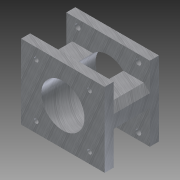
# Autodesk Inventor part: motor bracket GL-15N
Saved by Autodesk Inventor 2011 (Build 150239000, 239)
## iProperties
Created: 2014-01-21
Part Number: motor bracket GL-15N
Document SubType Name: Modeling
Designer: Devon
Density: 1 g/cm^3
Author: Devon
Autodesk Inventor part; units mm, degrees
ref_plane "YZ Plane" through (0, 0, 0) normal (1, 0, 0) x (0, 1, 0)
ref_plane "XZ Plane" through (0, 0, 0) normal (0, 1, 0) x (-1, 0, 0)
ref_plane "XY Plane" through (0, 0, 0) normal (0, 0, 1) x (1, 0, 0)
sketch "Sketch1" plane through (0, 0, 0) normal (0, 0, 1) x (1, 0, 0)
  line L0 (0, 0) -> (74, 0)
  line L1 (74, 0) -> (74, 66)
  line L2 (74, 66) -> (0, 66)
  line L3 (0, 66) -> (0, 0)
  line L4 (0, 0) -> (0, 9.43)
  line L5 (74, 0) -> (64.57, 0)
  line L6 (0, 66) -> (9.43, 66)
  line L7 (74, 66) -> (64.57, 66)
  line L8 (37, 33) -> (75, 33) construction
  line L9 (37, 33) -> (75, 33) construction
  circle A0 centre (10.1299, 59.8701) radius 2.5
  circle A1 centre (63.8701, 59.8701) radius 2.5
  circle A2 centre (63.8701, 6.1299) radius 2.5
  circle A3 centre (10.1299, 6.1299) radius 2.5
  dimension "d0" = 74
  dimension "d1" = 66
  dimension "d2" = 9.43
  dimension "d4" = 9.43
  dimension "d6" = 9.43
  dimension "d8" = 9.43
  dimension "d14" = 5
  dimension "d15" = 5
  dimension "d16" = 5
  dimension "d17" = 5
  constraints: 20 end point, 4 centre point, 4 point on line, 3 horizontal, 2 parallel, 1 perpendicular
  measures "d0" distance of L2.end L1.end
  measures "d1" distance of L1.end L0.end
  measures "d2" distance of L0.start L4.end
  measures "d4" distance of L0.end L5.end
  measures "d6" distance of L2.end L6.end
  measures "d8" distance of L1.end L7.end
  measures "d14" diameter of A0
  measures "d15" diameter of A1
  measures "d16" diameter of A2
  measures "d17" diameter of A3
extrude "Extrusion1" add sketch "Sketch1" along normal blind 8
sketch "Sketch2" plane through (0, 0, 8) normal (0, 0, 1) x (1, 0, 0)
  line L0 (0, 0) -> (0, 66) projected
  line L1 (74, 0) -> (0, 0) projected
  line L2 (74, 66) -> (74, 0) projected
  line L3 (5.4025, 46.4704) -> (0, 41.0679)
  line L4 (14.4661, 10.4661) -> (24.9321, 0)
  line L5 (68.5975, 46.4704) -> (74, 41.0679)
  line L6 (14.4661, 10.4661) -> (0, 24.9321)
  arc A0 (23.5296, 46.4704) -> (50.4704, 46.4704) centre (37, 33) ccw
  line L7 (50.4704, 46.4704) -> (68.5975, 46.4704)
  line L8 (23.5296, 46.4704) -> (5.4025, 46.4704)
  circle A1 centre (63.8701, 6.1299) radius 2.5 projected
  circle A2 centre (10.1299, 6.1299) radius 2.5 projected
  line L9 (57.1349, 12.8651) -> (74, 29.7303)
  line L10 (57.1349, 12.8651) -> (44.2697, 0)
  line L11 (10.1299, 6.1299) -> (16.8651, 12.8651)
  line L12 (16.8651, 12.8651) -> (0, 29.7303)
  line L13 (16.8651, 12.8651) -> (29.7303, 0)
  point P0 (49.0679, 0)
  point P1 (74, 24.9321)
  dimension "d23" = 38.1
  dimension "d26" = 9.525
  dimension "d27" = 9.525
  constraints: 22 end point, 10 point on line, 3 collinear, 2 perpendicular, 2 point on circle, 1 centre point
  measures "d23" diameter of A0
  measures "d26" distance of A1.centre L9.start
  measures "d27" distance of L11.start L11.end
extrude "Extrusion2" add sketch "Sketch2" along normal blind 32 contours L0 L3 L8 A0 L7 L5 L2 L9 L10 L1 L13 L12
sketch "Sketch4" plane through (0, 0, 40) normal (0, 0, 1) x (1, 0, 0)
  line L0 (0, 0) -> (74, 0)
  line L1 (74, 0) -> (74, 65.908)
  line L2 (74, 65.908) -> (0, 65.908)
  line L3 (0, 65.908) -> (0, 0)
  line L4 (4, 65.908) -> (70, 65.908)
  line L5 (70, 0) -> (4, 0)
  line L6 (4, 65.908) -> (13.43, 65.908)
  line L7 (13.43, 65.908) -> (13.43, 56.478)
  line L8 (4, 9.43) -> (13.43, 9.43)
  line L9 (70, 0) -> (60.57, 0)
  line L10 (60.57, 0) -> (60.57, 9.43)
  line L11 (70, 65.908) -> (60.57, 65.908)
  line L12 (60.57, 65.908) -> (60.57, 56.478)
  circle A0 centre (13.43, 56.478) radius 2
  circle A1 centre (13.43, 9.43) radius 2
  circle A2 centre (60.57, 9.43) radius 2
  circle A3 centre (60.57, 56.478) radius 2
  dimension "d30" = 9.43
  dimension "d31" = 9.43
  dimension "d32" = 9.43
  dimension "d33" = 9.43
  dimension "d34" = 9.43
  dimension "d35" = 9.43
  dimension "d36" = 9.43
  dimension "d37" = 9.43
  dimension "d38" = 4
  dimension "d39" = 4
  dimension "d40" = 4
  dimension "d41" = 4
  constraints: 26 end point, 4 centre point, 4 coincident, 4 perpendicular, 3 parallel, 3 point on line, 2 horizontal
  measures "d30" distance of L4.start L6.end
  measures "d31" distance of L6.end L7.end
  measures "d32" distance of L5.end L8.start
  measures "d33" distance of L8.start L8.end
  measures "d34" distance of L5.start L9.end
  measures "d35" distance of L9.end L10.end
  measures "d36" distance of L4.end L11.end
  measures "d37" distance of L11.end L12.end
  measures "d38" diameter of A0
  measures "d39" diameter of A1
  measures "d40" diameter of A2
  measures "d41" diameter of A3
extrude "Extrusion3" add sketch "Sketch4" along normal blind 8
sketch "Sketch5" plane through (0, 0, 48) normal (0, 0, 1) x (1, 0, 0)
  line L0 (0, 65.908) -> (74, 0)
  line L1 (74, 65.908) -> (0, 0)
  circle A0 centre (37, 32.954) radius 19.05
  dimension "d44" = 38.1
  constraints: 4 end point, 1 centre point, 1 midpoint
  measures "d44" diameter of A0
hole "Hole1" at (37, 32.954, 48) direction (0, 0, -1) diameter 38.1 depth 127 tip angle 118
body "Solid1"
